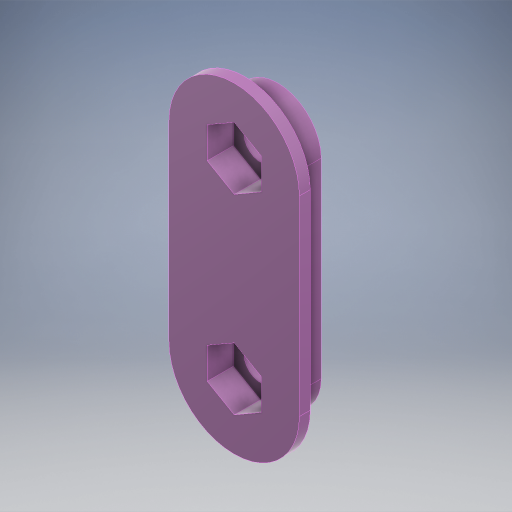
# Autodesk Inventor part: Нижний крепёж оснований
Saved by Autodesk Inventor 2023 (Build 270158000, 158)
## iProperties
Created: 2023-03-26
Part Number: Нижний крепёж оснований
Material: Типовые
Document SubType Name: Modeling
Designer: Admin
Density: 1 g/cm^3
Appearance: По умолчанию
Author: Admin
Autodesk Inventor part; units mm, degrees
ref_plane "YZ Plane" through (0, 0, 0) normal (1, 0, 0) x (0, 1, 0)
ref_plane "XZ Plane" through (0, 0, 0) normal (0, 1, 0) x (-1, 0, 0)
ref_plane "XY Plane" through (0, 0, 0) normal (0, 0, 1) x (1, 0, 0)
sketch "Эскиз1" plane through (0, 0, 0) normal (0, 0, 1) x (1, 0, 0)
  circle A0 centre (0, -17.5) radius 3
  line L0 (0, 23.2158) -> (4.95, 20.3579)
  arc A1 (11.95, 17.5) -> (-11.95, 17.5) centre (0, 17.5) ccw
  line L1 (4.95, 20.3579) -> (4.95, 14.6421)
  arc A2 (7.95, 17.5) -> (-7.95, 17.5) centre (0, 17.5) ccw
  line L2 (4.95, 14.6421) -> (0, 11.7842)
  circle A3 centre (0, 17.5) radius 3
  circle A4 centre (0, 17.5) radius 5.11
  line L3 (-4.95, 14.6421) -> (-4.95, 20.3579)
  line L4 (0, 11.7842) -> (-4.95, 14.6421)
  line L5 (-4.95, 20.3579) -> (0, 23.2158)
  line L6 (-11.95, -17.5) -> (-11.95, 17.5)
  line L7 (-7.95, 17.5) -> (-7.95, -17.5)
  line L8 (0, -17.5) -> (0, 17.5)
  line L9 (7.95, -17.5) -> (7.95, 17.5)
  line L10 (11.95, 17.5) -> (11.95, -17.5)
  arc A5 (-11.95, -17.5) -> (11.95, -17.5) centre (0, -17.5) ccw
  circle A6 centre (0, -17.5) radius 5.11
  arc A7 (-7.95, -17.5) -> (7.95, -17.5) centre (0, -17.5) ccw
  line L11 (4.95, -14.6421) -> (4.95, -20.3579)
  line L12 (4.95, -20.3579) -> (0, -23.2158)
  line L13 (0, -23.2158) -> (-4.95, -20.3579)
  line L14 (-4.95, -20.3579) -> (-4.95, -14.6421)
  line L15 (-4.95, -14.6421) -> (0, -11.7842)
  line L16 (0, -11.7842) -> (4.95, -14.6421)
  point P0 (0, 0)
  point P1 (0, 0)
  dimension "d0" = 6
  dimension "d1" = 10.22
  dimension "d2" = 4
  dimension "d3" = 6
  dimension "d5" = 35
  dimension "d12" = 7.95
  constraints: 36 end point, 8 centre point, 8 coincident, 8 point on circle, 4 tangent, 3 parallel, 3 vertical, 1 equal length, 1 equal radius, 1 midpoint, 29 other
  measures "d0" diameter of A3
  measures "d1" diameter of A4
  measures "d2" distance between parallel lines of L10 L9
  measures "d3" diameter of A0
  measures "d5" distance of L10.start L10.end
  measures "d12" radius of A2
extrude "Выдавливание1" add sketch "Эскиз1" along normal blind 2 contours A0 | L0 A4 L5 | A4 L0 | L0 A4 L1 L2 L4 L3 L5 | L5 A4 | L0 L1 A4 | A4 L3 L5 | A4 L1 | L3 A4 | L1 L2 A4 | A4 L4 L3 | A4 L2 | L4 A4 | L2 L8 A4 | A4 L8 L4 | L10 A5 L6 A1 | L9 A7 L7 A2 | A3 | A6 L15 L8 | L8 L16 A6 | A6 L16 L11 L12 L13 L14 L15 | A6 L16 | L15 A6 | L16 L11 A6 | A6 L14 L15 | A6 L11 | L14 A6 | L11 L12 A6 | A6 L13 L14 | A6 L12 | L13 A6 | L12 L13 A6
extrude "Выдавливание3" add sketch "Эскиз1" against normal blind 6 contours A0 | L0 A4 L5 | A4 L0 | L0 A4 L1 L2 L4 L3 L5 | L5 A4 | L0 L1 A4 | A4 L3 L5 | A4 L1 | L3 A4 | L1 L2 A4 | A4 L4 L3 | A4 L2 | L4 A4 | L2 L8 A4 | A4 L8 L4 | L9 A7 L7 A2 | A3 | A6 L15 L8 | L8 L16 A6 | A6 L16 L11 L12 L13 L14 L15 | A6 L16 | L15 A6 | L16 L11 A6 | A6 L14 L15 | A6 L11 | L14 A6 | L11 L12 A6 | A6 L13 L14 | A6 L12 | L13 A6 | L12 L13 A6
extrude "Выдавливание4" cut sketch "Эскиз1" along normal through all both and the other way through all contours A0 | A3
extrude "Выдавливание5" cut sketch "Эскиз1" along normal blind 2 and the other way blind 2.8 contours A0 | L0 A4 L5 | L0 A4 L1 L2 L4 L3 L5 | L0 L1 A4 | A4 L3 L5 | L1 L2 A4 | A4 L4 L3 | L2 L8 A4 | A4 L8 L4 | A3 | A6 L15 L8 | L8 L16 A6 | A6 L16 L11 L12 L13 L14 L15 | L16 L11 A6 | A6 L14 L15 | L11 L12 A6 | A6 L13 L14 | L12 L13 A6
